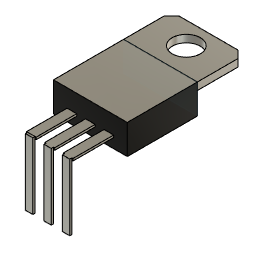
lm317 v1 (Autodesk Fusion 360 design; units mm, degrees)
Autodesk Fusion 360 part; units mm, degrees
sketch "Sketch1" plane through (0, 0, 0) normal (0, 1, 0) x (1, 0, 0)
  line L0 (0, 0) -> (10, 0)
  line L1 (10, 0) -> (10, -4)
  line L2 (10, -4) -> (0, -4)
  line L3 (0, -4) -> (0, 0)
  dimension "d1" = 10
  dimension "d2" = 4
  constraint horizontal L0
  constraint vertical L1
  constraint horizontal L2
  constraint vertical L3
  constraint coincident L0.start L3.end
  measures "d1" distance of L0.start L0.end
  measures "d2" distance of L0.start L2.end
extrude "Extrude1" add sketch "Sketch1" along normal blind 9.5 makes body 1
sketch "Sketch2" plane through (0, 0, 0) normal (0, 1, 0) x (1, 0, 0)
  line L0 (8.15, -1.3) -> (6.85, -1.3)
  line L1 (6.85, -1.3) -> (6.85, -1.6)
  line L2 (6.85, -1.6) -> (8.15, -1.6)
  line L3 (8.15, -1.6) -> (8.15, -1.3)
  line L4 (5.65, -1.3) -> (4.35, -1.3)
  line L5 (5.65, -1.6) -> (5.65, -1.3)
  line L6 (4.35, -1.6) -> (5.65, -1.6)
  line L7 (4.35, -1.3) -> (4.35, -1.6)
  line L8 (3.15, -1.3) -> (1.85, -1.3)
  line L9 (3.15, -1.6) -> (3.15, -1.3)
  line L10 (1.85, -1.6) -> (3.15, -1.6)
  line L11 (1.85, -1.3) -> (1.85, -1.6)
  dimension "d7" = 1.3
  dimension "d8" = 0.3
  dimension "d11" = -5
  dimension "d12" = 0
  constraint horizontal L0
  constraint vertical L1
  constraint horizontal L2
  constraint vertical L3
  measures "d7" distance of L0.start L0.end
  measures "d8" distance of L0.start L2.end
extrude "Extrude2" add sketch "Sketch2" against normal blind 5.5 bodies 1
sketch "Sketch3" plane through (0, 0, 0) normal (1, 0, 0) x (0, 1, 0)
  line L0 (-5.5, 1.6) -> (-5.8, 1.6)
  line L1 (-5.8, 1.6) -> (-5.8, -7.4)
  line L2 (-5.8, -7.4) -> (-5.5, -7.4)
  line L3 (-5.5, -7.4) -> (-5.5, 1.6)
  dimension "d15" = 0.3
  dimension "d16" = 9
  constraint horizontal L0
  constraint vertical L1
  constraint horizontal L2
  constraint vertical L3
  measures "d15" distance of L0.start L0.end
  measures "d16" distance of L0.start L2.end
extrude "Extrude3" add sketch "Sketch3" along normal blind 1 separate body makes body 2
move_face "MoveFace1" by (2.2, 0, 0) 1 faces at (0.3333, -5.8, -1.4) on bodies 2
move_body "Move1" bodies 2 to x (1, 0, 0) y (0, 1, 0) z (0, 0, 1) at (2, 0, 0)
sketch "Sketch4" plane through (0, -5.8, 0) normal (0, -1, 0) x (1, 0, 0)
  line L0 (2, 1.6) -> (2, -7.4)
  line L1 (2, -7.4) -> (3, -7.4)
  line L2 (3, -7.4) -> (3, 1.6)
  line L3 (3, 1.6) -> (2, 1.6)
  line L4 (5.5, 1.6) -> (4.5, 1.6)
  line L5 (4.5, 1.6) -> (4.5, -7.4)
  line L6 (5.5, -7.4) -> (5.5, 1.6)
  line L7 (4.5, -7.4) -> (5.5, -7.4)
  line L8 (8, 1.6) -> (7, 1.6)
  line L9 (7, 1.6) -> (7, -7.4)
  line L10 (8, -7.4) -> (8, 1.6)
  line L11 (7, -7.4) -> (8, -7.4)
  dimension "d21" = 5
  dimension "d22" = 0
extrude "Extrude4" add sketch "Sketch4" against normal blind 0.3 contours L4 L5 L6 L7 | L8 L9 L10 L11 bodies 1
sketch "Sketch5" plane through (0, 9.5, 0) normal (0, 1, 0) x (-1, 0, 0)
  line L0 (0, 4) -> (-10, 4)
  line L1 (-10, 4) -> (-10, 0)
  line L2 (-10, 0) -> (0, 0)
  line L3 (0, 0) -> (0, 4)
copy_body "Body->Comp1" bodies 1 removing the originals makes body 3 in component "Component"
copy_body "Body->Comp2" bodies 2 removing the originals makes body 4 in component "Component'"
sketch "Sketch6" plane through (0, 9.5, 0) normal (0, 1, 0) x (-1, 0, 0)
  line L0 (-10, 4) -> (0, 4)
  line L1 (0, 4) -> (0, 3)
  line L2 (0, 3) -> (-10, 3)
  line L3 (-10, 3) -> (-10, 4)
  constraint horizontal L0
  constraint vertical L1
  constraint horizontal L2
  constraint vertical L3
extrude "Extrude1'" add sketch "Sketch6" along normal blind 6.5 separate body makes body 5 in component "Component''"
sketch "Sketch7" plane through (0, 0, 4) normal (0, 0, 1) x (-1, 0, 0)
  line L0 (0, -9.5) -> (-10, -9.5)
  line L1 (-10, -9.5) -> (-10, -16)
  line L2 (-10, -16) -> (0, -16)
  line L3 (0, -16) -> (0, -9.5)
  circle A0 centre (-5, -13) radius 1.9
  dimension "d27" = 3.8
  measures "d27" diameter of A0
extrude "Extrude2'" cut sketch "Sketch7" against normal blind 1 contours A0 bodies 5 in component "Component''"
sketch "Sketch8" plane through (0, 0, 3) normal (0, 0, -1) x (1, 0, 0)
  circle A0 centre (5, -13) radius 1.9
  line L0 (10, -9.5) -> (0, -9.5)
  line L1 (0, -9.5) -> (0, -16)
  line L2 (0, -16) -> (10, -16)
  line L3 (10, -16) -> (10, -9.5)
  line L4 (0, -16) -> (0, -15)
  line L5 (0, -16) -> (1, -16)
  line L6 (1, -16) -> (0, -15)
  constraint coincident L1.end L2.start
  constraint coincident L1 L4.end
  constraint perpendicular L2 L4
  constraint coincident L2 L5.end
extrude "Extrude3'" cut sketch "Sketch8" against normal blind 1 contours L1 L2 L4 L5 L6 bodies 5 in component "Component''"
sketch "Sketch9" plane through (0, 0, 3) normal (0, 0, -1) x (1, 0, 0)
  line L0 (0, -15) -> (1, -16)
  line L1 (1, -16) -> (10, -16)
  line L2 (10, -16) -> (10, -9.5)
  line L3 (10, -9.5) -> (0, -9.5)
  line L4 (0, -9.5) -> (0, -15)
  circle A0 centre (5, -13) radius 1.9
  line L5 (10, -16) -> (9, -16)
  line L6 (10, -16) -> (10, -15)
  line L7 (10, -15) -> (9, -16)
  constraint coincident L1.end L2.start
  constraint coincident L1 L5.end
  constraint perpendicular L2 L5
  constraint coincident L2 L6.end
  constraint perpendicular L1 L6
extrude "Extrude4'" cut sketch "Sketch9" against normal blind 1 contours L1 L2 L5 L6 L7 bodies 5 in component "Component''"
component "Component" placed x (1, 0, 0) y (0, 1, 0) z (0, 0, 1) at (0, 0, 0)
component "Component'" placed x (1, 0, 0) y (0, 1, 0) z (0, 0, 1) at (0, 0, 0)
component "Component''" placed x (1, 0, 0) y (0, 1, 0) z (0, 0, 1) at (0, 0, 0)
